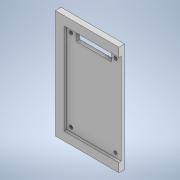
# Autodesk Inventor part: 2020-04-12 KeypadOnly
Saved by Autodesk Inventor 2020 (Build 240168000, 168)
## iProperties
Created: 2020-04-12
Part Number: 2020-04-12 KeypadOnly
Material: Generic
Document SubType Name: Modeling
Designer: torto
Density: 1 g/cm^3
Appearance: Default
Author: torto
Autodesk Inventor part; units mm, degrees
ref_plane "YZ Plane" through (0, 0, 0) normal (1, 0, 0) x (0, 1, 0)
ref_plane "XZ Plane" through (0, 0, 0) normal (0, 1, 0) x (-1, 0, 0)
ref_plane "XY Plane" through (0, 0, 0) normal (0, 0, 1) x (1, 0, 0)
sketch "Sketch1" plane through (0, 0, 0) normal (0, 0, 1) x (1, 0, 0)
  line L0 (-28.08, -48.025) -> (28.08, -48.025)
  line L1 (28.08, -48.025) -> (28.08, 48.025)
  line L2 (28.08, 48.025) -> (-28.08, 48.025)
  line L3 (-28.08, 48.025) -> (-28.08, -48.025)
  line L4 (-28.08, -48.025) -> (28.08, 48.025) construction
  line L5 (28.08, -48.025) -> (-28.08, 48.025) construction
  point P0 (0, 0)
  dimension "Length" = 56.16
  dimension "Height" = 96.05
  constraints: 3 horizontal, 2 end point, 2 vertical alignment, 15 other
  measures "Length" distance of point (28.08, 48.025) point (-28.08, 48.025)
  measures "Height" distance of L0.end point (28.08, 48.025)
extrude "BasicShape" add sketch "Sketch1" along normal blind 5
sketch "KeypadDimensions" plane through (0, 0, 5) normal (0, 0, 1) x (1, 0, 0)
  line L0 (-28.08, -48.025) -> (28.08, -48.025) construction
  line L1 (28.08, -48.025) -> (3.93, -48.025) construction
  line L2 (3.93, -48.025) -> (3.93, 0) construction
  line L3 (3.93, 0) -> (28.08, 0) construction
  line L4 (28.08, 0) -> (28.08, -48.025) construction
  line L5 (-20.22, -40.2) -> (28.08, -40.2)
  line L6 (28.08, -40.2) -> (28.08, 40.2)
  line L7 (28.08, 40.2) -> (-20.22, 40.2)
  line L8 (-20.22, 40.2) -> (-20.22, -40.2)
  line L9 (-20.22, -40.2) -> (28.08, 40.2) construction
  line L10 (28.08, -40.2) -> (-20.22, 40.2) construction
  point P0 (0, 0)
  dimension "d4" = 24.15
  dimension "d5" = 48.025
  dimension "KeypadLength" = 48.3
  dimension "KeypadHeight" = 80.4
  constraints: 20 end point, 4 parallel, 2 horizontal, 2 midpoint, 2 perpendicular
  measures "d4" distance of L2.end L3.end
  measures "d5" distance of L1.end L2.end
  measures "KeypadLength" distance of L7.end L6.end
  measures "KeypadHeight" distance of L7.end L5.start
extrude "KeypadCountersink" cut sketch "KeypadDimensions" against normal blind 2
sketch "Sketch3" plane through (0, 0, 3) normal (0, 0, 1) x (1, 0, 0)
  line L0 (-20.22, -40.2) -> (-20.22, 40.2) projected
  line L1 (-20.22, 40.2) -> (-11.72, 40.2)
  line L2 (-11.72, 40.2) -> (-11.72, 31.7)
  line L3 (-11.72, 31.7) -> (-20.22, 31.7)
  line L4 (-20.22, 31.7) -> (-20.22, 40.2)
  line L5 (-20.22, 40.2) -> (28.08, 40.2) projected
  line L6 (28.08, 40.2) -> (19.58, 40.2)
  line L7 (19.58, 40.2) -> (19.58, 31.7)
  line L8 (19.58, 31.7) -> (28.08, 31.7)
  line L9 (28.08, 31.7) -> (28.08, 40.2)
  line L10 (28.08, -40.2) -> (-20.22, -40.2) projected
  line L11 (-20.22, -40.2) -> (-11.72, -40.2)
  line L12 (-11.72, -40.2) -> (-11.72, -31.7)
  line L13 (-11.72, -31.7) -> (-20.22, -31.7)
  line L14 (-20.22, -31.7) -> (-20.22, -40.2)
  line L15 (28.08, -40.2) -> (19.58, -40.2)
  line L16 (19.58, -40.2) -> (19.58, -31.7)
  line L17 (19.58, -31.7) -> (28.08, -31.7)
  line L18 (28.08, -31.7) -> (28.08, -40.2)
  line L19 (-11.72, 31.7) -> (19.58, 31.7)
  line L20 (-20.22, 40.2) -> (-16.27, 40.2) construction
  line L21 (-16.27, 40.2) -> (-16.27, 35.95) construction
  line L22 (-16.27, 35.95) -> (-20.22, 35.95) construction
  line L23 (-20.22, 35.95) -> (-20.22, 40.2) construction
  circle A0 centre (-16.27, 35.95) radius 1.75 construction
  circle A1 centre (-16.27, 35.95) radius 1.5
  line L24 (28.08, 40.2) -> (28.08, -40.2) construction
  line L25 (28.08, 40.2) -> (23.13, 40.2) construction
  line L26 (23.13, 40.2) -> (23.13, 35.95) construction
  line L27 (23.13, 35.95) -> (28.08, 35.95) construction
  line L28 (28.08, 35.95) -> (28.08, 40.2) construction
  circle A2 centre (23.13, 35.95) radius 1.5
  line L29 (28.08, -40.2) -> (23.13, -40.2) construction
  line L30 (23.13, -40.2) -> (23.13, -36.25) construction
  line L31 (23.13, -36.25) -> (28.08, -36.25) construction
  line L32 (28.08, -36.25) -> (28.08, -40.2) construction
  line L33 (-20.22, -40.2) -> (-16.27, -40.2) construction
  line L34 (-16.27, -40.2) -> (-16.27, -36.25) construction
  line L35 (-16.27, -36.25) -> (-20.22, -36.25) construction
  line L36 (-20.22, -36.25) -> (-20.22, -40.2) construction
  circle A3 centre (-16.27, -36.25) radius 1.5
  circle A4 centre (23.13, -36.25) radius 1.5
  point P0 (0, 0)
  dimension "d10" = 8.5
  dimension "d11" = 8.5
  dimension "d12" = 8.5
  dimension "d13" = 8.5
  dimension "CornerLength" = 8.5
  dimension "d15" = 8.5
  dimension "d16" = 8.5
  dimension "d17" = 8.5
  dimension "KeypadHoleDiameter" = 3.5
  dimension "KeypadScrewHoleDiameterUntapped" = 3
  dimension "UpperKeypadHoleSpacingY" = 4.25
  dimension "LeftKeypadHoleSpacingX" = 3.95
  dimension "RightKeypadHoleSpacingX" = 4.95
  dimension "d23" = 4.25
  dimension "d25" = 3
  dimension "d26" = 4.95
  dimension "LowerKeypadHoleSpacingY" = 3.95
  dimension "d28" = 3
  dimension "d29" = 3
  dimension "d30" = 3.95
  dimension "d31" = 3.95
  constraints: 66 end point, 16 parallel, 8 horizontal, 8 perpendicular, 5 centre point, 5 coincident
  measures "d10" distance of L2.end L3.end
  measures "d11" distance of L1.end L2.end
  measures "d12" distance of L8.end L7.end
  measures "d13" distance of L7.end L6.end
  measures "CornerLength" distance of L13.end L12.end
  measures "d15" distance of L12.end L11.end
  measures "d16" distance of L16.end L17.end
  measures "d17" distance of L15.end L16.end
  measures "KeypadHoleDiameter" diameter of A0
  measures "KeypadScrewHoleDiameterUntapped" diameter of A1
  measures "UpperKeypadHoleSpacingY" distance of L20.end L21.end
  measures "LeftKeypadHoleSpacingX" distance of L21.end L22.end
  measures "RightKeypadHoleSpacingX" distance of L26.end L27.end
  measures "d23" distance of L25.end L26.end
  measures "d25" diameter of A2
  measures "d26" distance of L30.end L31.end
  measures "LowerKeypadHoleSpacingY" distance of L29.end L30.end
  measures "d28" diameter of A4
  measures "d29" diameter of A3
  measures "d30" distance of L33.end L34.end
  measures "d31" distance of L34.end L35.end
extrude "Extrusion3" cut sketch "Sketch3" against normal blind 5 contours L2 L5 L7 L19 | A1 | A2 | A3 | A4
thread "Thread1" size "M3x0.5" class "6H" standard "ANSI Metric M Profile" length 5
thread "Thread2" size "M3x0.5" class "6H" standard "ANSI Metric M Profile" length 5
thread "Thread3" size "M3x0.5" class "6H" standard "ANSI Metric M Profile" length 5
thread "Thread4" size "M3x0.5" class "6H" standard "ANSI Metric M Profile" length 3
equation "\"d4\" = 0.5 * KeypadLength"
equation "\"d5\" = 0.5 * Height"
equation "\"d15\" = CornerLength"
equation "\"d16\" = CornerLength"
equation "\"d17\" = CornerLength"
equation "\"d23\" = UpperKeypadHoleSpacingY"
equation "\"d25\" = KeypadScrewHoleDiameterUntapped"
equation "\"d26\" = RightKeypadHoleSpacingX"
equation "\"d28\" = KeypadScrewHoleDiameterUntapped"
equation "\"d29\" = KeypadScrewHoleDiameterUntapped"
equation "\"d30\" = LowerKeypadHoleSpacingY"
equation "\"d31\" = LeftKeypadHoleSpacingX"
equation "\"d32\" = Thickness"
equation "\"d34\" = Thickness"
equation "\"d36\" = Thickness"
equation "\"d38\" = Thickness"
equation "\"Thickness\" = 5"
body "Solid1"
